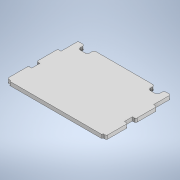
# Autodesk Inventor part: back_wall
Saved by Autodesk Inventor 2020 (Build 240168000, 168)
## iProperties
Created: 2019-06-12
Part Number: back_wall
Material: Generic
Document SubType Name: Modeling
Designer: Dammy
Density: 1 g/cm^3
Appearance: Default
Author: Dammy
Autodesk Inventor part; units mm, degrees
ref_plane "YZ Plane" through (0, 0, 0) normal (1, 0, 0) x (0, 1, 0)
ref_plane "XZ Plane" through (0, 0, 0) normal (0, 1, 0) x (-1, 0, 0)
ref_plane "XY Plane" through (0, 0, 0) normal (0, 0, 1) x (1, 0, 0)
sketch "Sketch1" plane through (0, 0, 0) normal (0, 1, 0) x (-1, 0, 0)
  line L0 (-2, -70.675) -> (-4.5, -70.675)
  line L1 (-4.5, -41.675) -> (-2, -41.675)
  line L2 (0, -43.675) -> (0, -68.675)
  line L3 (-4.5, -30.675) -> (-2, -30.675)
  line L4 (0, -28.675) -> (0, -3.675)
  line L5 (-2, -1.675) -> (-4.5, -1.675)
  arc A0 (0, -3.675) -> (-2, -1.675) centre (-2, -3.675) ccw
  arc A1 (-2, -30.675) -> (0, -28.675) centre (-2, -28.675) ccw
  arc A2 (0, -43.675) -> (-2, -41.675) centre (-2, -43.675) ccw
  arc A3 (-2, -70.675) -> (0, -68.675) centre (-2, -68.675) ccw
  line L6 (-133.5, -70.675) -> (-131, -70.675)
  line L7 (-131, -41.675) -> (-133.5, -41.675)
  line L8 (-135.5, -43.675) -> (-135.5, -68.675)
  line L9 (-133.5, -30.675) -> (-131, -30.675)
  line L10 (-131, -1.675) -> (-133.5, -1.675)
  line L11 (-135.5, -3.675) -> (-135.5, -28.675)
  arc A4 (-133.5, -1.675) -> (-135.5, -3.675) centre (-133.5, -3.675) ccw
  arc A5 (-135.5, -28.675) -> (-133.5, -30.675) centre (-133.5, -28.675) ccw
  arc A6 (-133.5, -41.675) -> (-135.5, -43.675) centre (-133.5, -43.675) ccw
  arc A7 (-135.5, -68.675) -> (-133.5, -70.675) centre (-133.5, -68.675) ccw
  line L12 (-26.25, -91) -> (-26.25, -88)
  line L13 (-109.25, -91) -> (-109.25, -88)
  line L14 (-29.25, -94) -> (-106.25, -94)
  line L15 (0, -56.175) -> (-135.5, -56.175) construction
  line L16 (-112.25, -85) -> (-118.95, -85)
  line L17 (-121.95, -88) -> (-121.95, -91)
  line L18 (-124.95, -94) -> (-129.2679, -94)
  line L19 (-23.25, -85) -> (-16.55, -85)
  line L20 (-13.55, -88) -> (-13.55, -91)
  line L21 (-10.55, -94) -> (-6.5, -94)
  arc A8 (-13.55, -91) -> (-10.55, -94) centre (-10.55, -91) ccw
  arc A9 (-13.55, -88) -> (-16.55, -85) centre (-16.55, -88) ccw
  arc A10 (-23.25, -85) -> (-26.25, -88) centre (-23.25, -88) ccw
  arc A11 (-29.25, -94) -> (-26.25, -91) centre (-29.25, -91) ccw
  arc A12 (-109.25, -91) -> (-106.25, -94) centre (-106.25, -91) ccw
  arc A13 (-109.25, -88) -> (-112.25, -85) centre (-112.25, -88) ccw
  arc A14 (-118.95, -85) -> (-121.95, -88) centre (-118.95, -88) ccw
  arc A15 (-124.95, -94) -> (-121.95, -91) centre (-124.95, -91) ccw
  line L22 (-7.5, 0) -> (-128.9984, 0)
  line L23 (-4.5, -70.675) -> (-4.5, -92)
  line L24 (-4.5, -30.675) -> (-4.5, -41.675)
  line L25 (-131, -30.675) -> (-131, -41.675)
  line L26 (-131, -70.675) -> (-131, -91)
  line L27 (-128.9984, 0) -> (-130, 0)
  line L28 (-131, -1) -> (-131, -1.675)
  arc A16 (-130, 0) -> (-131, -1) centre (-130, -1) ccw
  line L29 (-4.5, -1.675) -> (-4.5, -1)
  line L30 (-4.5, 0) -> (-4.5, 0)
  line L31 (-5.5, 0) -> (-7.5, 0)
  arc A17 (-4.5, -1) -> (-5.5, 0) centre (-5.5, -1) ccw
  line L32 (-131, -91) -> (-131, -92)
  line L33 (-129, -94) -> (-127.109, -94)
  arc A18 (-131, -92) -> (-129, -94) centre (-129, -92) ccw
  line L34 (-4.5, -94) -> (-8.525, -94)
  arc A19 (-6.5, -94) -> (-4.5, -92) centre (-6.5, -92) ccw
  point P0 (0, 0)
  point P1 (0, -70.675)
  point P2 (-3.25, -70.675)
  point P3 (-135.5, -41.675)
  point P4 (-135.5, -30.675)
  point P5 (-132.25, -70.675)
  point P6 (-131, -94)
  point P7 (-26.25, -94)
  point P8 (-26.25, -85)
  point P9 (-109.25, -94)
  point P10 (-109.25, -85)
  point P11 (-67.75, -94)
  point P12 (-67.75, -56.175)
  point P13 (-121.95, -85)
  point P14 (-13.55, -85)
  point P15 (-6.4873, -94)
  point P16 (-4.5, -91.775)
  point P17 (-3.25, -1.675)
  point P18 (-132.25, -1.675)
  point P19 (0, -16.175)
  point P20 (-4.5, -81.3375)
  point P21 (-4.5, -36.175)
  point P22 (-131, -80.8375)
  point P23 (-131, -36.175)
  point P24 (-135.5, -16.175)
  point P25 (-131, -1.3375)
  dimension "d3" = 4.5
  dimension "d8" = 2
  dimension "d11" = 2
  dimension "d12" = 2
  dimension "d13" = 9
  dimension "d14" = 83
  dimension "d15" = 12.7
  dimension "d16" = 12.7
  dimension "d18" = 3
  dimension "d19" = 3
  dimension "d20" = 135.5
  dimension "d23" = 94.0001
  dimension "d24" = 4.5
  dimension "d25" = 1
  dimension "d26" = 1
  dimension "d29" = 29
  dimension "d30" = 23.325
  dimension "d31" = 2
  dimension "d32" = 69
  dimension "d33" = 11
  dimension "d34" = 2
  constraints: 70 end point, 40 point on circle, 40 tangent, 28 point on line, 20 centre point, 17 midpoint, 13 vertical alignment, 11 equal radius, 9 horizontal, 9 horizontal alignment, 6 parallel, 6 perpendicular, 6 vertical, 3 collinear
  measures "d3" distance of point (0, -70.675) L0.end
  measures "d8" radius of A0
  measures "d11" radius of A4
  measures "d12" radius of A6
  measures "d13" distance of point (-26.25, -94) point (-26.25, -85)
  measures "d14" distance between parallel lines of L13 L12
  measures "d15" distance of point (-109.25, -85) point (-121.95, -85)
  measures "d16" distance of point (-26.25, -85) point (-13.55, -85)
  measures "d18" radius of A8
  measures "d19" radius of A12
  measures "d20" distance of L15.start L15.end
  measures "d23" distance between parallel lines of L22 L14
  measures "d24" distance between parallel lines of L8 L26
  measures "d25" radius of A16
  measures "d26" radius of A17
  measures "d29" distance from line of L1 point (-3.25, -70.675)
  measures "d30" distance from line of L21 point (-3.25, -70.675)
  measures "d31" radius of A18
  measures "d32" distance between parallel lines of L5 L0
  measures "d33" distance between parallel lines of L3 L1
  measures "d34" radius of A19
extrude "Extrusion1" add sketch "Sketch1" along normal blind 5
equation "\"d19\" = d18"
equation "\"d24\" = d3"
equation "\"d25\" = d26"
equation "\"d31\" = d17"
equation "\"d33\" = d32 - 2 * d29"
equation "\"d17\" = 2"
body "Solid1"
